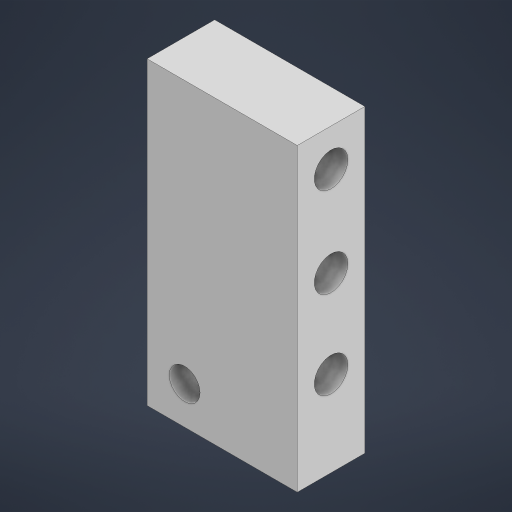
# Autodesk Inventor part: Torsion_Spring_Lift
Saved by Autodesk Inventor 2023 (Build 270158000, 158)
## iProperties
Created: 2024-02-27
Part Number: Torsion_Spring_Lift
Material: Generic
Document SubType Name: Modeling
Designer: kelle
Density: 1 g/cm^3
Appearance: Default
Author: kelle
Autodesk Inventor part; units mm, degrees
ref_plane "YZ Plane" through (0, 0, 0) normal (1, 0, 0) x (0, 1, 0)
ref_plane "XZ Plane" through (0, 0, 0) normal (0, 1, 0) x (-1, 0, 0)
ref_plane "XY Plane" through (0, 0, 0) normal (0, 0, 1) x (1, 0, 0)
sketch "Sketch1" plane through (0, 0, 0) normal (0, 0, 1) x (1, 0, 0)
  line L0 (12.7, -25.4) -> (-12.7, -25.4)
  line L1 (-12.7, -25.4) -> (-12.7, 25.4)
  line L2 (-12.7, 25.4) -> (12.7, 25.4)
  line L3 (12.7, 25.4) -> (12.7, -25.4)
  line L4 (12.7, -25.4) -> (-12.7, 25.4) construction
  line L5 (-12.7, -25.4) -> (12.7, 25.4) construction
  line L6 (-12.7, 25.4) -> (0, 25.4)
  circle A0 centre (-6.35, -19.05) radius 2.6035
  line L7 (-12.7, 25.4) -> (-3.7, 25.4) construction
  line L8 (-3.7, 25.4) -> (-3.7, -25.4) construction
  line L9 (-3.7, -25.4) -> (-12.7, -25.4) construction
  line L10 (-12.7, -25.4) -> (-12.7, 25.4) construction
  point P0 (0, 0)
  dimension "d0" = 25.4
  dimension "d1" = 50.8
  dimension "d4" = 5.207
  dimension "d5" = 6.35
  dimension "d7" = 9
  dimension "d8" = 6.35
  constraints: 22 end point, 4 parallel, 3 horizontal, 2 midpoint, 2 perpendicular, 1 centre point, 1 point on line
  measures "d0" distance of L1.end L2.end
  measures "d1" distance of L0.end L1.end
  measures "d4" diameter of A0
  measures "d5" distance from line of L1 A0.centre
  measures "d7" distance of L8.end L9.end
  measures "d8" distance from line of L0 A0.centre
extrude "Extrusion1" add sketch "Sketch1" along normal blind 11.43
sketch "Sketch2" plane through (-12.7, -25.4, 0) normal (-1, 0, 0) x (0, 0, 1)
  line L0 (0, 50.8) -> (0, 0) projected
  line L1 (0, 0) -> (11.43, 0) projected
  line L2 (11.43, 50.8) -> (11.43, 0) projected
  line L3 (0, 50.8) -> (11.43, 50.8) projected
  line L4 (0, 50.8) -> (11.43, 50.8) construction
  line L5 (5.715, 50.8) -> (5.715, 0) construction
  line L6 (0, 0) -> (11.43, 0) construction
  line L7 (0, 25.4) -> (11.43, 25.4) construction
  line L8 (11.43, 0) -> (11.43, 50.8) construction
  circle A0 centre (5.715, 44.45) radius 2.85
  circle A1 centre (5.715, 29.2354) radius 2.85
  circle A2 centre (5.715, 14.4018) radius 2.85
  dimension "d11" = 5.7
  dimension "d12" = 6.35
  dimension "d13" = 5.7
  dimension "d14" = 15.2146
  dimension "d15" = 5.7
  dimension "d16" = 14.8336
  constraints: 4 end point, 3 centre point, 3 midpoint, 3 point on line
  measures "d11" diameter of A0
  measures "d12" distance from line of L3 A0.centre
  measures "d13" diameter of A1
  measures "d14" distance of A0.centre A1.centre
  measures "d15" diameter of A2
  measures "d16" distance of A1.centre A2.centre
extrude "Extrusion2" cut sketch "Sketch2" against normal blind 9 contours A0 | A1 | A2
sketch "Sketch3" plane through (12.7, -25.4, 0) normal (1, 0, 0) x (0, 0, -1)
  line L0 (0, 0) -> (0, 50.8) projected
  line L1 (0, 50.8) -> (-11.43, 50.8) projected
  line L2 (-11.43, 0) -> (-11.43, 50.8) projected
  line L3 (0, 0) -> (-11.43, 0) projected
  circle A0 centre (-5.715, 44.45) radius 2.85 projected
  circle A1 centre (-5.715, 29.2354) radius 2.85 projected
  circle A2 centre (-5.715, 14.4018) radius 2.85 projected
  point P0 (0, 25.4)
extrude "Extrusion3" cut sketch "Sketch3" against normal blind 9 contours A0 | A1 | A2
body "Solid1"
